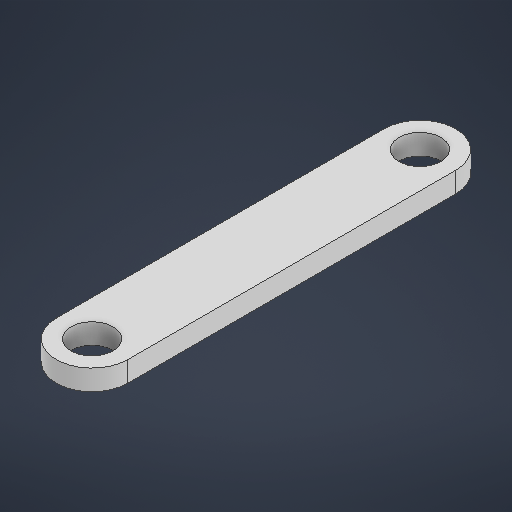
# Autodesk Inventor part: Micro_servo_frame_1
Saved by Autodesk Inventor 2026.1 (Build 301233020, 233B)
## iProperties
Created: 2025-10-15
Part Number: Micro_servo_frame_1
Material: Generic
Document SubType Name: Modeling
Designer: Asus
Density: 1 g/cm^3
Appearance: Default
Author: Asus
Autodesk Inventor part; units mm, degrees
ref_plane "YZ Plane" through (0, 0, 0) normal (1, 0, 0) x (0, 1, 0)
ref_plane "XZ Plane" through (0, 0, 0) normal (0, 1, 0) x (-1, 0, 0)
ref_plane "XY Plane" through (0, 0, 0) normal (0, 0, 1) x (1, 0, 0)
sketch "Sketch1" plane through (0, 0, 0) normal (0, 1, 0) x (-1, 0, 0)
  circle A0 centre (0, 0) radius 2.05
  circle A1 centre (0, -32) radius 2.05
  line L0 (0, 0) -> (0, -32) construction
  line L1 (-3.5, 0) -> (-3.5, -32)
  line L2 (3.5, -32) -> (3.5, 0)
  arc A2 (3.5, 0) -> (-3.5, 0) centre (0, 0) ccw
  arc A3 (-3.5, -32) -> (3.5, -32) centre (0, -32) ccw
  point P0 (0, -16)
  dimension "d1" = 4.1
  dimension "d2" = 4.1
  dimension "d3" = 7
  constraints: 8 end point, 4 centre point, 4 point on circle, 4 tangent, 1 coincident, 1 midpoint, 1 parallel
  measures "d1" diameter of A0
  measures "d2" diameter of A1
  measures "d3" diameter of A3
extrude "Extrusion1" add sketch "Sketch1" along normal blind 2
body "Solid1"
